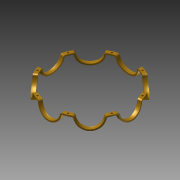
# Autodesk Inventor part: Curea
Saved by Autodesk Inventor 2011 SP2 (Build 150309200, 309)
## iProperties
Created: 2023-03-13
Part Number: Curea
Document SubType Name: Modeling
Designer: utilizator
Density: 1 g/cm^3
Author: utilizator
Autodesk Inventor part; units mm, degrees
ref_plane "YZ Plane" through (0, 0, 0) normal (1, 0, 0) x (0, 1, 0)
ref_plane "XZ Plane" through (0, 0, 0) normal (0, 1, 0) x (-1, 0, 0)
ref_plane "XY Plane" through (0, 0, 0) normal (0, 0, 1) x (1, 0, 0)
sketch "Sketch1" plane through (0, 0, 0) normal (0, 0, 1) x (1, 0, 0)
  circle A0 centre (0, 0) radius 47
  circle A1 centre (0, 0) radius 43
  dimension "d0" = 47
  dimension "d1" = 43
  constraints: 2 centre point, 2 coincident
  measures "d0" radius of A0
  measures "d1" radius of A1
extrude "Extrusion1" add sketch "Sketch1" along normal blind 16
sketch "Sketch2" plane through (0, 0, 16) normal (0, 0, 1) x (1, 0, 0)
  circle A0 centre (0, 0) radius 43 projected
  circle A1 centre (0, 0) radius 47 projected
  circle A2 centre (0, 0) radius 45 construction
  line L0 (0, 57) -> (0, 33)
  arc A3 (0, 33) -> (0, 57) centre (0, 45) ccw
  dimension "d4" = 45
  dimension "d6" = 12
  dimension "d7" = 24
  constraints: 2 end point, 2 point on circle, 2 vertical alignment, 1 centre point, 1 coincident, 1 vertical, 2 other
  measures "d6" radius of A3
  measures "d7" distance of L0.start L0.end
revolve "Revolution1" cut sketch "Sketch2" angle 360 about axis through (0, 57, 16) along (0, -1, 0) picked at (2.1277, 39.698) picked at (9.2342, 44.2356) contours A3 L0 A0 | A0 L0 A1 A3 | A1 L0 A3
fillet "Fillet1" radius 2 2 edges at (-11.8958, 43.422, 16) (11.8958, 43.422, 16)
pattern_circular "Circular Pattern1" count 8 over 360 about axis through (0, 0, -10) along (0, 0, 1) of "Revolution1", "Fillet1"
shell "Shell1" thickness 1.5 removed faces 3 at (-42.8149, -19.3877, 9.1357) at (15.5416, -40.0931, 7.5887) at (-43.9397, 4.565, 0)
sketch "Sketch3" plane through (0, 0, 16) normal (0, 0, 1) x (1, 0, 0)
  arc A0 (19.5669, 38.2902) -> (13.2394, 40.9111) centre (0, 0) ccw projected
  line L0 (0, -65.8062) -> (0, 65.8062) projected
  circle A1 centre (0, 0) radius 45 construction
  line L1 (0, 0) -> (17.2208, 41.5746) construction
  circle A2 centre (17.2208, 41.5746) radius 1
  dimension "d14" = 45
  dimension "d15" = 22.5
  dimension "d16" = 1
  constraints: 2 coincident, 2 end point, 1 centre point, 3 other
  measures "d15" angle of L0 L1
  measures "d16" radius of A2
extrude "Extrusion2" cut sketch "Sketch3" against normal blind 16
pattern_circular "Circular Pattern2" count 8 over 360 about axis through (0, 0, -10) along (0, 0, 1) of "Extrusion2"
body "Solid1"
